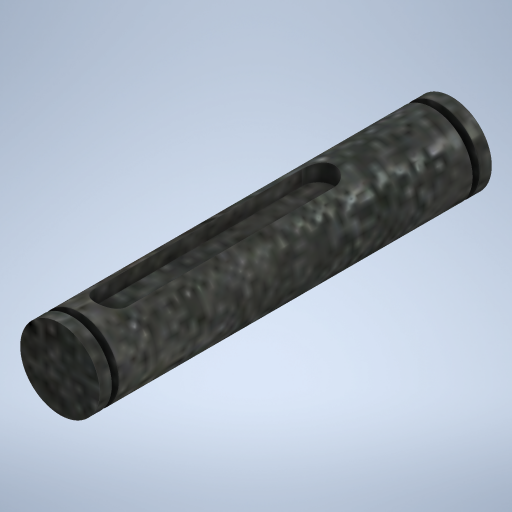
# Autodesk Inventor part: gearbox_shaft1
Saved by Autodesk Inventor 2023 (Build 270158000, 158)
## iProperties
Created: 2023-05-28
Part Number: gearbox_shaft1
Material: Steel
Document SubType Name: Modeling
Designer: 310611102
Density: 7.85 g/cm^3
Appearance: Plate
Mass: 27.6472 g
Surface Area: 19.1979 cm^2
Volume: 3.52194 cm^3
Vendor: 亞里士
Author: 310611102
Autodesk Inventor part; units mm, degrees
ref_plane "YZ Plane" through (0, 0, 0) normal (1, 0, 0) x (0, 1, 0)
ref_plane "XY Plane" through (0, 0, 0) normal (0, 0, 1) x (1, 0, 0)
sketch "Sketch5" plane through (0, 0, 0) normal (1, 0, 0) x (0, 1, 0)
  line L0 (0, 0) -> (5, 0)
  line L1 (5, 0) -> (5, -1.5)
  line L2 (5, -1.5) -> (3.55, -1.5)
  line L3 (3.55, -1.5) -> (3.55, -2.4)
  line L4 (3.55, -2.4) -> (5, -2.4)
  line L5 (5, -2.4) -> (5, -46.9)
  line L6 (5, -46.9) -> (3.55, -46.9)
  line L7 (3.55, -46.9) -> (3.55, -47.8)
  line L8 (3.55, -47.8) -> (5, -47.8)
  line L9 (5, -47.8) -> (5, -49.3)
  line L10 (5, -49.3) -> (0, -49.3)
  line L11 (0, -49.3) -> (0, 0)
  dimension "d14" = 49.3
  dimension "d15" = 10
  dimension "d16" = 1.5
  dimension "d17" = 0.9
  dimension "d18" = 7.1
  dimension "d19" = 1.5
  dimension "d20" = 0.9
  constraints: 24 end point, 8 perpendicular, 6 point on line, 1 horizontal
  measures "d14" distance of L10.end L0.start
  measures "d15" diameter of L9 L11
  measures "d16" distance of L8.end L9.end
  measures "d17" distance of L6.end L7.end
  measures "d18" diameter of L7 L11
  measures "d19" distance of L0.end L1.end
  measures "d20" distance of L2.end L3.end
revolve "Revolution1" add sketch "Sketch5" angle 360 about axis through (0, 0, -49.3) along (0, 0, 1)
ref_plane "Work Plane1" through (0, 5, 0) normal (0, 1, 0) x (-1, 0, 0)
sketch "Sketch6" plane through (0, 5, 0) normal (0, 1, 0) x (-1, 0, 0)
  line L0 (0, -6.5) -> (0, -32.5) construction
  line L1 (-2, -6.5) -> (-2, -32.5)
  line L2 (2, -32.5) -> (2, -6.5)
  arc A0 (2, -6.5) -> (-2, -6.5) centre (0, -6.5) ccw
  arc A1 (-2, -32.5) -> (2, -32.5) centre (0, -32.5) ccw
  line L3 (5, -1.5) -> (-5, -1.5) projected
  point P0 (0, 0)
  point P1 (0, -19.5)
  point P2 (0, -4.5)
  point P3 (0, -34.5)
  dimension "d23" = 4
  dimension "d24" = 30
  dimension "d25" = 3
  constraints: 8 end point, 6 point on circle, 4 tangent, 2 centre point, 1 midpoint, 1 parallel, 1 vertical, 1 vertical alignment
  measures "d23" distance between parallel lines of L1 L2
  measures "d24" distance of point (0, -4.5) point (0, -34.5)
  measures "d25" distance from line of L3 point (0, -4.5)
extrude "Extrusion4" cut sketch "Sketch6" against normal blind 2.3
body "Solid2"
